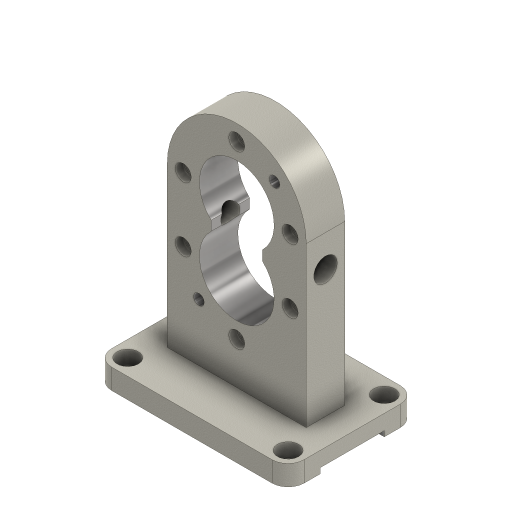
# Autodesk Inventor part: Part024. Bearing box
Saved by Autodesk Inventor 2023.2 (Build 272271030, 271C)
## iProperties
Created: 2023-10-05
Part Number: Part024. Bearing box
Material: Steel, Carbon
Document SubType Name: Modeling
Designer: User
Mass: 7361.8 g
Surface Area: 1343.53 cm^2
Volume: 937.809 cm^3
Density: 7.85 g/cm^3
Appearance: Steel - Cast
Author: User
Autodesk Inventor part; units mm, degrees
ref_plane "YZ Plane" through (0, 0, 0) normal (1, 0, 0) x (0, 1, 0)
ref_plane "XZ Plane" through (0, 0, 0) normal (0, 1, 0) x (-1, 0, 0)
sketch "Sketch1" plane through (0, 0, 0) normal (0, 1, 0) x (-1, 0, 0)
  line L0 (90, 60) -> (-90, 60)
  line L1 (-90, 60) -> (-90, -60)
  line L2 (-90, -60) -> (90, -60)
  line L3 (90, -60) -> (90, 60)
  line L4 (90, 60) -> (-90, -60) construction
  line L5 (-90, 60) -> (90, -60) construction
  point P0 (0, 0)
  dimension "d0" = 180
  dimension "d1" = 120
  constraints: 12 end point, 2 midpoint, 2 parallel, 1 horizontal, 1 perpendicular
  measures "d0" distance of L2.end L1.end
  measures "d1" distance of L1.end L0.end
extrude "Extrusion1" add sketch "Sketch1" along normal blind 19
fillet "Fillet1" radius 15 4 edges at (90, 9.5, 60) (90, 9.5, -60) (-90, 9.5, -60) (-90, 9.5, 60)
sketch "Sketch2" plane through (0, 0, 0) normal (0, 0, 1) x (1, 0, 0)
  line L0 (75, 19) -> (-75, 19) projected
  line L1 (-65, 19) -> (-65, 168)
  arc A0 (65, 168) -> (-65, 168) centre (0, 168) ccw
  line L2 (65, 168) -> (65, 19)
  line L3 (75, 0) -> (-75, 0) projected
  point P0 (0, 0)
  point P1 (0, 0)
  dimension "d5" = 168
  dimension "d6" = 65
  constraints: 4 end point, 2 point on circle, 2 point on line, 2 tangent, 1 centre point, 1 midpoint, 1 perpendicular, 1 vertical, 1 vertical alignment
  measures "d5" distance from line of L3 A0.centre
  measures "d6" radius of A0
extrude "Extrusion2" add sketch "Sketch2" along normal mid plane 36
sketch "Sketch3" plane through (0, 0, 18) normal (0, 0, 1) x (1, 0, 0)
  arc A0 (65, 168) -> (-65, 168) centre (0, 168) ccw projected
  arc A1 (24, 142.5245) -> (-24, 142.5245) centre (0, 168) ccw
  arc A2 (-24, 133.4755) -> (24, 133.4755) centre (0, 108) ccw
  line L0 (-24, 142.5245) -> (-24, 133.4755)
  line L1 (24, 142.5245) -> (24, 133.4755)
  point P0 (0, 0)
  dimension "d9" = 70
  dimension "d10" = 70
  dimension "d11" = 60
  dimension "d12" = 48
  constraints: 4 end point, 4 point on circle, 2 centre point, 2 parallel, 1 coincident, 1 vertical, 1 vertical alignment
  measures "d9" diameter of A1
  measures "d10" diameter of A2
  measures "d11" distance of A2.centre A0.centre
  measures "d12" distance between parallel lines of L1 L0
extrude "Extrusion3" cut sketch "Sketch3" along normal through all both and the other way through all
sketch "Sketch4" plane through (90, 0, 45) normal (1, 0, 0) x (0, 0, -1)
  line L0 (0, 0) -> (90, 0) projected
  line L1 (15, 0) -> (75, 0)
  line L2 (75, 0) -> (75, 5)
  line L3 (75, 5) -> (15, 5)
  line L4 (15, 5) -> (15, 0)
  line L5 (15, 0) -> (75, 5) construction
  line L6 (75, 0) -> (15, 5) construction
  point P0 (45, 0)
  point P1 (45, 2.5)
  point P2 (45, 0)
  dimension "d15" = 60
  dimension "d16" = 5
  constraints: 12 end point, 4 midpoint, 2 parallel, 1 horizontal, 1 perpendicular
  measures "d15" distance of L3.end L2.end
  measures "d16" distance of L2.end L1.end
extrude "Extrusion4" cut sketch "Sketch4" against normal through all
sketch "Sketch5" plane through (0, 0, 18) normal (0, 0, 1) x (1, 0, 0)
  arc A0 (24, 142.5245) -> (-24, 142.5245) centre (0, 168) ccw projected
  point P0 (0, 0)
  point P1 (50, 168)
  dimension "d19" = 50
  constraints: 1 horizontal alignment
  measures "d19" distance of point (50, 168) A0.centre
hole "Hole1" at (50, 168, 18) direction (0, 0, -1) diameter 12 end through all counterbore diameter 15 counterbore depth 8
sketch "Sketch6" plane through (0, 0, -18) normal (0, 0, -1) x (-1, 0, 0)
  circle A0 centre (-50, 168) radius 6 projected
  point P0 (0, 0)
  constraints: 1 coincident
hole "Hole2" at (50, 168, -18) direction (0, 0, 1) diameter 15 depth 8
pattern_circular "Circular Pattern1" count 3 over 180 about axis through (0, 168, 18) along (0, 0, 1) of "Hole1", "Hole2"
ref_plane "Work Plane1" through (-24, 138, 18) normal (0, 1, 0) x (1, 0, 0)
mirror "Mirror1" about plane through (-24, 138, 18) normal (0, 1, 0) of "Hole1", "Hole2", "Circular Pattern1"
sketch "Sketch7" plane through (0, 0, 18) normal (0, 0, 1) x (1, 0, 0)
  arc A0 (-24, 133.4755) -> (24, 133.4755) centre (0, 108) ccw projected
  arc A1 (65, 168) -> (-65, 168) centre (0, 168) ccw projected
  line L0 (0, 168) -> (35.3553, 203.3553) construction
  line L1 (0, 108) -> (-35.3553, 72.6447) construction
  line L2 (-126, 0) -> (126, 0) construction
  point P0 (0, 0)
  dimension "d37" = 50
  dimension "d38" = 45
  constraints: 4 end point, 2 parallel
  measures "d37" distance of L0.start L0.end
  measures "d38" angle of L2 L0
hole "Hole3" at (35.3553, 203.3553, 18) at (-35.3553, 72.6447, 18) direction (0, 0, -1) diameter 10 end through all
sketch "Sketch8" plane through (0, 19, 0) normal (0, 1, 0) x (1, 0, 0)
  arc A0 (-90, -45) -> (-75, -60) centre (-75, -45) ccw projected
  arc A1 (75, -60) -> (90, -45) centre (75, -45) ccw projected
  arc A2 (90, 45) -> (75, 60) centre (75, 45) ccw projected
  arc A3 (-75, 60) -> (-90, 45) centre (-75, 45) ccw projected
  point P0 (0, 0)
hole "Hole4" at (-75, 19, 45) at (75, 19, 45) at (75, 19, -45) at (-75, 19, -45) direction (0, -1, 0) diameter 15 end through all counterbore diameter 20 counterbore depth 13
sketch "Sketch9" plane through (65, 19, 18) normal (1, 0, 0) x (0, 0, -1)
  line L0 (0, 123.5245) -> (36, 123.5245) projected
  line L1 (36, 114.4755) -> (0, 114.4755) projected
  line L2 (36, 114.4755) -> (0, 114.4755) projected
  line L3 (36, 123.5245) -> (0, 114.4755)
  point P0 (18, -19)
  point P1 (18, 119)
  point P2 (18, 119)
  constraints: 2 end point, 1 coincident, 1 midpoint
hole "Hole5" at (65, 138, 0) direction (-1, 0, 0) diameter 18 depth 41 counterbore diameter 22 counterbore depth 15
mirror "Mirror2" about plane through (0, 0, 0) normal (1, 0, 0) of "Hole5"
ref_plane "Work Plane2" through (-24, 138, 18) normal (0, 1, 0) x (1, 0, 0)
body "Solid1"
